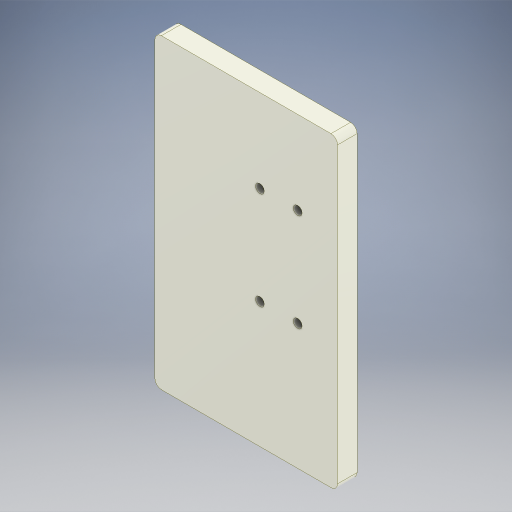
# Autodesk Inventor part: foot_ver2
Saved by Autodesk Inventor 2024 (Build 280153000, 153)
## iProperties
Created: 2024-09-04
Part Number: foot_ver2
Material: PMMA 플라스틱
Document SubType Name: Modeling
Designer: msi
Density: 1.188 g/cm^3
Appearance: 매끄러움 - 아이보리색
Author: msi
Autodesk Inventor part; units mm, degrees
ref_plane "YZ Plane" through (0, 0, 0) normal (1, 0, 0) x (0, 1, 0)
ref_plane "XZ Plane" through (0, 0, 0) normal (0, 1, 0) x (-1, 0, 0)
ref_plane "XY Plane" through (0, 0, 0) normal (0, 0, 1) x (1, 0, 0)
sketch "스케치1" plane through (0, 0, 0) normal (0, 0, 1) x (1, 0, 0)
  circle A0 centre (11, 3) radius 1.35 projected
  circle A1 centre (-5, 3) radius 1.35 projected
  line L0 (0, 0) -> (6, 0) projected
  line L1 (6, 0) -> (6, 6) projected
  line L2 (0, 6) -> (6, 6) projected
  line L3 (0, 0) -> (0, 6) projected
  circle A2 centre (11, -53.9) radius 1.35 projected
  circle A3 centre (-5, -53.9) radius 1.35 projected
  line L4 (0, -56.9) -> (6, -56.9) projected
  line L5 (6, -56.9) -> (6, -50.9) projected
  line L6 (0, -50.9) -> (6, -50.9) projected
  line L7 (0, -56.9) -> (0, -50.9) projected
  line L8 (21, 16) -> (-35, 16)
  line L9 (-35, 16) -> (-35, -78)
  line L10 (-35, -78) -> (21, -78)
  line L11 (21, -78) -> (21, 16)
  circle A4 centre (11, 3) radius 1.35
  circle A5 centre (-5, 3) radius 1.35
  circle A6 centre (11, -53.9) radius 1.35
  circle A7 centre (-5, -53.9) radius 1.35
  line L12 (-0.05, 6.05) -> (6.05, 6.05)
  line L13 (6.05, 6.05) -> (6.05, -0.05)
  line L14 (6.05, -0.05) -> (-0.05, -0.05)
  line L15 (-0.05, -0.05) -> (-0.05, 6.05)
  line L16 (-0.05, 6.05) -> (6.05, -0.05) construction
  line L17 (6.05, 6.05) -> (-0.05, -0.05) construction
  line L18 (-0.05, -50.85) -> (6.05, -50.85)
  line L19 (6.05, -50.85) -> (6.05, -56.95)
  line L20 (6.05, -56.95) -> (-0.05, -56.95)
  line L21 (-0.05, -56.95) -> (-0.05, -50.85)
  line L22 (-0.05, -50.85) -> (6.05, -56.95) construction
  line L23 (6.05, -50.85) -> (-0.05, -56.95) construction
  point P0 (3, 3)
  point P1 (3, -53.9)
  dimension "d0" = 56
  dimension "d1" = 94
  dimension "d2" = 2.7
  dimension "d3" = 2.7
  dimension "d4" = 2.7
  dimension "d5" = 2.7
  dimension "d6" = 6.1
  dimension "d7" = 6.1
  dimension "d8" = 6.1
  dimension "d9" = 6.1
  constraints: 32 end point, 6 parallel, 4 centre point, 4 coincident, 4 midpoint, 3 horizontal, 3 perpendicular
  measures "d0" distance of L10.end L9.end
  measures "d1" distance of L9.end L8.end
  measures "d2" diameter of A4
  measures "d3" diameter of A5
  measures "d4" diameter of A6
  measures "d5" diameter of A7
  measures "d6" distance of L13.end L14.end
  measures "d7" distance of L12.end L13.end
  measures "d8" distance of L19.end L20.end
  measures "d9" distance of L18.end L19.end
extrude "돌출1" add sketch "스케치1" along normal blind 6 contours L11 L10 L9 L8
fillet "모깎기1" radius 2 4 edges at (-35, 16, 3) (21, 16, 3) (-35, -78, 3) (21, -78, 3)
sketch "스케치3" plane through (0, 0, 6) normal (0, 0, 1) x (1, 0, 0)
  line L0 (-0.05, 6.05) -> (6.05, 6.05) projected
  line L1 (6.05, 6.05) -> (6.05, -0.05) projected
  line L2 (-0.05, -0.05) -> (-0.05, 6.05) projected
  line L3 (6.05, -0.05) -> (-0.05, -0.05) projected
  line L4 (-2.05, -0.05) -> (8.05, -0.05)
  line L5 (8.05, -0.05) -> (8.05, 6.05)
  line L6 (8.05, 6.05) -> (-2.05, 6.05)
  line L7 (-2.05, 6.05) -> (-2.05, -0.05)
  line L8 (-2.05, -0.05) -> (8.05, 6.05) construction
  line L9 (8.05, -0.05) -> (-2.05, 6.05) construction
  line L10 (-0.05, -50.85) -> (6.05, -50.85) projected
  line L11 (6.05, -50.85) -> (6.05, -56.95) projected
  line L12 (-0.05, -56.95) -> (-0.05, -50.85) projected
  line L13 (6.05, -56.95) -> (-0.05, -56.95) projected
  line L14 (-2.05, -56.95) -> (8.05, -56.95)
  line L15 (8.05, -56.95) -> (8.05, -50.85)
  line L16 (8.05, -50.85) -> (-2.05, -50.85)
  line L17 (-2.05, -50.85) -> (-2.05, -56.95)
  line L18 (-2.05, -56.95) -> (8.05, -50.85) construction
  line L19 (8.05, -56.95) -> (-2.05, -50.85) construction
  point P0 (0, 0)
  point P1 (3, 3)
  point P2 (3, -53.9)
  dimension "d13" = 10.1
  dimension "d14" = 10.1
  dimension "d15" = 6.1
  constraints: 24 end point, 4 midpoint, 4 parallel, 2 horizontal, 2 perpendicular
  measures "d13" distance of L6.end L5.end
  measures "d14" distance of L16.end L15.end
  measures "d15" distance of L15.end L14.end
extrude "돌출2" cut sketch "스케치3" against normal blind 10
sketch "스케치4" plane through (0, 0, 6) normal (0, 0, 1) x (1, 0, 0)
  line L0 (-2.05, 6.05) -> (8.05, 6.05) projected
  line L1 (8.05, 6.05) -> (8.05, -0.05) projected
  line L2 (-2.05, -0.05) -> (-2.05, 6.05) projected
  line L3 (8.05, -0.05) -> (-2.05, -0.05) projected
  line L4 (-2.05, -50.85) -> (8.05, -50.85) projected
  line L5 (8.05, -50.85) -> (8.05, -56.95) projected
  line L6 (8.05, -56.95) -> (-2.05, -56.95) projected
  line L7 (-2.05, -56.95) -> (-2.05, -50.85) projected
  circle A0 centre (-2.05, 6.05) radius 1
  circle A1 centre (8.05, 6.05) radius 1
  circle A2 centre (8.05, -0.05) radius 1
  circle A3 centre (-2.05, -0.05) radius 1
  circle A4 centre (-2.05, -50.85) radius 1
  circle A5 centre (8.05, -50.85) radius 1
  circle A6 centre (8.05, -56.95) radius 1
  circle A7 centre (-2.05, -56.95) radius 1
  point P0 (0, 0)
  dimension "d18" = 2
  dimension "d19" = 2
  dimension "d20" = 2
  dimension "d21" = 2
  dimension "d22" = 2
  dimension "d23" = 2
  dimension "d24" = 2
  dimension "d25" = 2
  constraints: 8 centre point, 8 coincident
  measures "d18" diameter of A0
  measures "d19" diameter of A1
  measures "d20" diameter of A2
  measures "d21" diameter of A3
  measures "d22" diameter of A4
  measures "d23" diameter of A5
  measures "d24" diameter of A6
  measures "d25" diameter of A7
extrude "돌출3" cut sketch "스케치4" against normal blind 10 contours L2 A0 L0 | L0 A0 L2 | A1 L1 L0 | L0 L1 A1 | A3 L3 L2 | L2 L3 A3 | A2 L3 L1 | L1 L3 A2 | L7 A4 L4 | L4 A4 L7 | A5 L5 L4 | L4 L5 A5 | A7 L6 L7 | L7 L6 A7 | A6 L6 L5 | L5 L6 A6
sketch "스케치5" plane through (0, 0, 6) normal (0, 0, 1) x (1, 0, 0)
  line L0 (-1.05, 6.05) -> (7.05, 6.05) projected
  line L1 (8.05, 5.05) -> (8.05, 0.95) projected
  circle A0 centre (-2.8, -9.5) radius 1.35
  circle A1 centre (8.8, -9.5) radius 1.35
  circle A2 centre (-2.8, -39.5) radius 1.35
  circle A3 centre (8.8, -39.5) radius 1.35
  point P0 (0, 0)
  dimension "d32" = 2.7
  dimension "d33" = 2.7
  dimension "d34" = 2.7
  dimension "d35" = 2.7
  constraints: 4 centre point
  measures "d32" diameter of A0
  measures "d33" diameter of A1
  measures "d34" diameter of A2
  measures "d35" diameter of A3
extrude "돌출4" cut sketch "스케치5" against normal blind 10
sketch "스케치6" plane through (0, 0, 6) normal (0, 0, 1) x (1, 0, 0)
  line L0 (-11.1766, 9.439) -> (14.0881, 9.439)
  line L1 (14.0881, 9.439) -> (14.0881, -4.9308)
  line L2 (14.0881, -4.9308) -> (-11.1766, -4.9308)
  line L3 (-11.1766, -4.9308) -> (-11.1766, 9.439)
  line L4 (-9.3673, -48.6772) -> (15.6068, -48.6772)
  line L5 (15.6068, -48.6772) -> (15.6068, -64.9024)
  line L6 (15.6068, -64.9024) -> (-9.3673, -64.9024)
  line L7 (-9.3673, -64.9024) -> (-9.3673, -48.6772)
  point P0 (0, 0)
  constraints: 16 end point, 4 parallel, 2 horizontal, 2 perpendicular
extrude "돌출5" add sketch "스케치6" against normal blind 6
